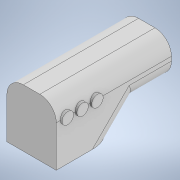
# Autodesk Inventor part: Weapon-Electric-Body
Saved by Autodesk Inventor 2020 (Build 240168000, 168)
## iProperties
Created: 2019-11-14
Part Number: Weapon-Electric-Body
Material: Generic
Document SubType Name: Modeling
Designer: vifly_01
Density: 1 g/cm^3
Appearance: Default
Author: vifly_01
Autodesk Inventor part; units mm, degrees
ref_plane "YZ Plane" through (0, 0, 0) normal (1, 0, 0) x (0, 1, 0)
ref_plane "XZ Plane" through (0, 0, 0) normal (0, 1, 0) x (-1, 0, 0)
ref_plane "XY Plane" through (0, 0, 0) normal (0, 0, 1) x (1, 0, 0)
sketch "Sketch1" plane through (0, 0, 0) normal (0, 0, 1) x (1, 0, 0)
  line L0 (7.5, -8.75) -> (-7.5, -8.75)
  line L1 (-7.5, -8.75) -> (-7.5, 8.75)
  line L2 (-7.5, 8.75) -> (7.5, 8.75)
  line L3 (7.5, 8.75) -> (7.5, -8.75)
  line L4 (7.5, -8.75) -> (-7.5, 8.75) construction
  line L5 (-7.5, -8.75) -> (7.5, 8.75) construction
  point P0 (0, 0)
  dimension "d0" = 15
  dimension "d1" = 17.5
  constraints: 12 end point, 2 midpoint, 2 parallel, 1 horizontal, 1 perpendicular
  measures "d0" distance of L1.end L2.end
  measures "d1" distance of L0.end L1.end
extrude "Extrusion1" add sketch "Sketch1" along normal blind 35
sketch "Sketch2" plane through (7.5, -8.75, 0) normal (1, 0, 0) x (0, 0, -1)
  line L0 (0, 0) -> (-35, 0) projected
  line L1 (-17.0033, 0) -> (-10.7814, 6.2327)
  line L2 (-10.7814, 6.2327) -> (0, 6.2327)
  line L3 (0, 6.2327) -> (0, 0)
  line L4 (0, 0) -> (-17.0033, 0)
  point P0 (0, 8.75)
  constraints: 8 end point, 2 perpendicular, 1 parallel, 1 point on line
extrude "Extrusion2" cut sketch "Sketch2" against normal blind 35
fillet "Fillet3" radius 5 6 edges at (7.5, 8.75, 17.5) (7.5, -2.5173, 5.3907) (7.5, -5.6336, 13.8924) (-7.5, -5.6336, 13.8924) (-7.5, -2.5173, 5.3907) (-7.5, 8.75, 17.5)
sketch "Sketch3" plane through (0, 0, 0) normal (1, 0, 0) x (0, 1, 0)
  line L0 (3.75, 0) -> (3.75, 35) projected
  circle A0 centre (3.75, 32) radius 1.75
  point P0 (0, 0)
  point P1 (3.75, 33.75)
  point P2 (3.75, 30.25)
  dimension "d9" = 3.5
  constraints: 1 centre point, 1 point on line
  measures "d9" diameter of A0
extrude "Extrusion3" add sketch "Sketch3" along normal blind 8
pattern_linear "Rectangular Pattern1" count 3 spacing 4.5 along (0, 0, -1) of "Extrusion3"
body "Solid1"
